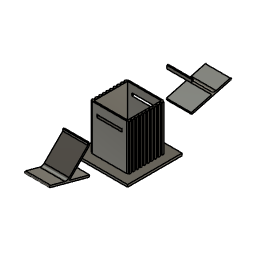
stojanek_complete (Autodesk Fusion 360 design; units mm, degrees)
Autodesk Fusion 360 part; units mm, degrees
sketch "Sketch1" plane through (0, 0, 0) normal (0, 0, 1) x (1, 0, 0)
  line L0 (60, 60) -> (-60, 60)
  line L1 (-60, 60) -> (-60, -60)
  line L2 (-60, -60) -> (60, -60)
  line L3 (60, -60) -> (60, 60)
  line L4 (60, 60) -> (-60, -60) construction
  line L5 (-60, 60) -> (60, -60) construction
  dimension "d1" = 120
  dimension "d60" = 120
  constraint horizontal L0
  constraint perpendicular L0 L1
  constraint parallel L0 L2
  constraint parallel L1 L3
  constraint coincident L4 origin
  constraint coincident L5 origin
  measures "d1" distance of L1.end L2.end
  measures "d60" distance of L0.end L1.end
extrude "Extrude1" add sketch "Sketch1" along normal blind 5 makes body 1
sketch "Sketch2" plane through (0, 0, 5) normal (0, 0, 1) x (-1, 0, 0)
  line L0 (-60, 60) -> (-60, -60)
  line L1 (-60, -60) -> (60, -60)
  line L2 (60, -60) -> (60, 60)
  line L3 (60, 60) -> (-60, 60)
  line L4 (-40, -40) -> (40, -40)
  line L5 (40, -40) -> (40, 40)
  line L6 (40, 40) -> (-40, 40)
  line L7 (-40, 40) -> (-40, -40)
  line L8 (-40, -40) -> (40, 40) construction
  line L9 (40, -40) -> (-40, 40) construction
  line L10 (60, 60) -> (-60, 60)
  line L11 (-60, 60) -> (-60, -60)
  dimension "d5" = 80
  dimension "d6" = 80
  dimension "d61" = 20
  dimension "d62" = 20
  constraint horizontal L4
  constraint perpendicular L4 L5
  constraint parallel L4 L6
  constraint parallel L5 L7
  constraint coincident L8 origin
  constraint coincident L9 origin
  measures "d5" distance of L5.end L6.end
  measures "d6" distance of L4.end L5.end
  measures "d61" distance of L6 L10
  measures "d62" distance of L7 L11
extrude "Extrude2" add sketch "Sketch2" along normal blind 100 contours L4 L5 L6 L7 bodies 1
shell "Shell1" thickness 3 removed faces 1 at (13.3333, -13.3333, 105) on bodies 1
sketch "Sketch7" plane through (0, 0, 0) normal (1, 0, 0) x (0, 1, 0)
  line L0 (-40, 5) -> (40, 5)
  line L1 (40, 105) -> (-40, 105)
  line L2 (-40, 105) -> (-40, 5)
  point P0 (37, 105)
  point P1 (0, 105)
  constraint midpoint L1 P1
sketch "Sketch8" plane through (0, 0, 0) normal (1, 0, 0) x (0, 1, 0)
  line L0 (58.7892, 102) -> (58.7892, 97.6569)
  line L1 (58.7892, 97.6569) -> (103.7892, 52.6569)
  line L2 (103.7892, 52.6569) -> (142.4262, 63.0096)
  line L3 (55.7892, 95) -> (99.3278, 51.4614)
  line L4 (142.4262, 63.0096) -> (143.4615, 59.1459)
  line L5 (58.7892, 102) -> (55.7892, 102)
  line L6 (55.7892, 102) -> (55.7892, 95)
  line L7 (143.4615, 59.1459) -> (55.7728, 35.6498)
  line L8 (99.3278, 51.4614) -> (54.7375, 39.5135)
  line L9 (54.7375, 39.5135) -> (55.7728, 35.6498)
  point P0 (37, 105)
  dimension "d72" = 135
  dimension "d73" = 45
  dimension "d74" = 40
  dimension "d88" = 3
  dimension "d90" = 4
  dimension "d91" = 4
  dimension "d116" = 120
  dimension "d121" = 60
  dimension "d124" = 87.6887
  dimension "d125" = 90
  dimension "d127" = 90
  dimension "d128" = 90
  dimension "d129" = 20
  dimension "d136" = 7
  dimension "d137" = 3
  constraint vertical L0
  constraint perpendicular L7 L9
  constraint coincident L3 L8.start
  constraint coincident L4.end L7.start
  measures "d72" angle of L0 L1
  measures "d73" horizontal distance of L0.end L1.end
  measures "d74" distance of L1.end L2.end
  measures "d88" distance of L0 L5.end
  measures "d90" distance of L2.end L4.end
  measures "d116" angle of L1 L2
  measures "d121" angle of L3 L8
  measures "d124" horizontal distance of L4.end L7.end
  measures "d125" angle of L2 L4
  measures "d127" angle of L5 L6
  measures "d128" angle of L0 L5
  measures "d129" distance of origin L7
  measures "d136" distance of L3.start L5.end
  measures "d137" distance of L5 P0
extrude "Extrude11" add sketch "Sketch8" along normal mid plane 55 bodies 1 makes body 2
sketch "Sketch9" plane through (0, 0, 5) normal (0, 0, 1) x (-1, 0, 0)
copy_body "CopyPasteBodies1" bodies 2 makes body 3
ref_plane "WorkPlane1" through (0, 42, 54) normal (0, -1, 0) x (1, 0, 0)
sketch "Sketch14" plane through (0, 42, 0) normal (0, -1, 0) x (-1, 0, 0)
combine "Combine4" operation add target body 3 tool bodies 2
move_body "Move3" bodies 3 to x (1, 0, 0) y (0, 1, 0) z (0, 0, 1) at (0, -31.789, 0)
ref_plane "WorkPlane3" through (0, 0, 55) normal (0, -1, 0) x (1, 0, 0)
mirror "Mirror2" about plane through (0, 0, 55) normal (0, -1, 0) of bodies 3 makes body 4
combine "Combine6" operation cut target body 1 tool bodies 4 3 keep tools
split "Split5" by plane through (0, 0, 5) normal (0, 0, 1) bodies 1 makes body 5 at (40, 12.3333, 71.6667)
fillet "Fillet7" radius 10 1 edges at (0, 72.0002, 52.6569) on bodies 3 4
fillet "Fillet7" radius 10 1 edges at (0, -72.0002, 52.6569) on bodies 3 4
sketch "Sketch16" plane through (40, 0, 0) normal (1, 0, 0) x (0, 1, 0)
  line L0 (-40, 5) -> (40, 5)
  line L1 (40, 5) -> (40, 105)
  line L2 (40, 105) -> (-40, 105)
  line L3 (-40, 105) -> (-40, 5)
  line L4 (-38, 105) -> (-34, 105)
  line L5 (-34, 105) -> (-34, 5)
  line L6 (-34, 5) -> (-38, 5)
  line L7 (-38, 5) -> (-38, 105)
  dimension "d142" = 2
  dimension "d143" = 4
  constraint horizontal L4
  constraint vertical L5
  constraint horizontal L6
  constraint vertical L7
  constraint coincident L0 L5.end
  constraint coincident L2 L4.start
  measures "d142" distance of L3 L7
  measures "d143" distance of L4.start L4.end
extrude "Extrude16" add sketch "Sketch16" along normal blind 2 contours L0 L2 L4 L5 L6 L7 bodies 1 5
pattern_linear "R-Pattern5" count 10 spacing 8 along (0, 1, 0) of "Extrude16"
sketch "Sketch17" plane through (-40, 0, 0) normal (-1, 0, 0) x (0, -1, 0)
  line L0 (-40, 5) -> (40, 5)
  line L1 (40, 5) -> (40, 105)
  line L2 (40, 105) -> (-40, 105)
  line L3 (-40, 105) -> (-40, 5)
  line L4 (-38, 105) -> (-34, 105)
  line L5 (-34, 105) -> (-34, 5)
  line L6 (-34, 5) -> (-38, 5)
  line L7 (-38, 5) -> (-38, 105)
  dimension "d150" = 2
  dimension "d151" = 4
  constraint horizontal L4
  constraint vertical L5
  constraint horizontal L6
  constraint vertical L7
  constraint coincident L0 L5.end
  constraint coincident L2 L4.start
  measures "d150" distance of L3 L7
  measures "d151" distance of L4.start L4.end
extrude "Extrude17" add sketch "Sketch17" along normal blind 2 contours L0 L2 L4 L5 L6 L7 bodies 1
pattern_linear "R-Pattern6" count 10 spacing 8 along (0, -1, 0) of "Extrude17"
fillet "Fillet8" radius 2 4 edges at (40, 40, 55) (40, -40, 55) (-40, -40, 55) (-40, 40, 55) on bodies 1
fillet "Fillet9" radius 2 2 edges at (0, 110.6372, 63.0096) (0, 111.6725, 59.1459) on bodies 3
fillet "Fillet10" radius 2 2 edges at (0, -110.6372, 63.0096) (0, -111.6725, 59.1459) on bodies 4
extrude "Extrude18" cut 1 faces at (9.1667, -38, 81.0002) along direction (0, 0.707107, -0.707107) blind 0.1 on bodies 1 bodies 1
extrude "Extrude19" cut 1 faces at (-27.5, -38, 84.7243) along direction (-1, 0, 0) blind 0.1 on bodies 1 bodies 1
extrude "Extrude20" cut 1 faces at (27.5, -38, 84.7243) along direction (1, 0, 0) blind 0.1 on bodies 1 bodies 1
extrude "Extrude21" cut 1 faces at (9.2, -38, 86.657) along direction (0, -0.707107, 0.707107) blind 0.1 on bodies 1 bodies 1
extrude "Extrude22" cut 1 faces at (9.1667, -39, 39.6734) along direction (0, -0.258819, -0.965926) blind 0.1 on bodies 1 bodies 1
extrude "Extrude23" cut 1 faces at (-27.5, -39, 42.3996) along direction (-1, 0, 0) blind 0.1 on bodies 1 bodies 1
extrude "Extrude24" cut 1 faces at (27.5, -39, 42.3996) along direction (1, 0, 0) blind 0.1 on bodies 1 bodies 1
extrude "Extrude25" cut 1 faces at (-9.1667, 38, 81.0002) along direction (0, -0.707107, -0.707107) blind 0.1 on bodies 1 bodies 1
extrude "Extrude26" cut 1 faces at (-27.5, 38, 84.7243) along direction (-1, 0, 0) blind 0.1 on bodies 1 bodies 1
extrude "Extrude27" cut 1 faces at (27.5, 38, 84.7243) along direction (1, 0, 0) blind 0.1 on bodies 1 bodies 1
extrude "Extrude28" cut 1 faces at (-9.2, 38, 86.657) along direction (0, 0.707107, 0.707107) blind 0.1 on bodies 1 bodies 1
extrude "Extrude29" cut 1 faces at (-9.1667, 39, 43.8145) along direction (0, -0.258819, 0.965926) blind 0.1 on bodies 1 bodies 1
extrude "Extrude30" cut 1 faces at (9.1667, 39, 39.6734) along direction (0, 0.258819, -0.965926) blind 0.1 on bodies 1 bodies 1
extrude "Extrude31" cut 1 faces at (-27.5, 38, 40.7858) along direction (-1, 0, 0) blind 0.1 on bodies 1 bodies 1
extrude "Extrude32" cut 1 faces at (27.5, 38, 40.7858) along direction (1, 0, 0) blind 0.1 on bodies 1 bodies 1
extrude "Extrude33" cut 1 faces at (9.2, -38, 43.5465) along direction (0, 0.258819, 0.965926) blind 0.1 on bodies 1 bodies 1
move_body "Move4" bodies 4 to x (1, 0, 0) y (0, 1, 0) z (0, 0, 1) at (0, -8.2237, -6.6793)
move_body "Move5" bodies 3 to x (1, 0, 0) y (0, 1, 0) z (0, 0, 1) at (0, 90, 0)
move_body "Move6" bodies 4 to x (1, 0, 0) y (0, 1, 0) z (0, 0, 1) at (0, -80, 0)
delete_face "DeleteFace6" 4 faces at (9.2, 39.0086, 39.5722) (27.6, 38, 40.7858) (-9.2, 37.9914, 43.6478) (-27.6, 38, 40.7858) on bodies 1
delete_face "DeleteFace7" 4 faces at (-9.2, -38.9827, 43.9134) (-9.2, -39.0086, 39.5722) (27.6, -38, 40.7858) (-27.6, -38, 40.7858) on bodies 1
equation "d124 = 95.6887414112 mm - 8 mm"
named bodies: "platform", "Right", "Left", "main"
